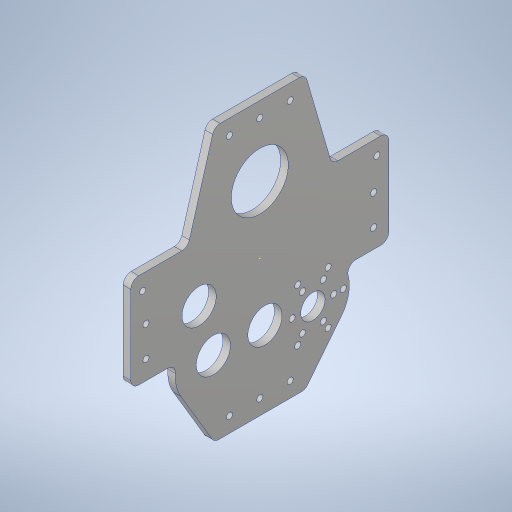
# Autodesk Inventor part: EL2-CGB-001
Saved by Autodesk Inventor 2023.4 (Build 274418000, 418)
## iProperties
Created: 2025-01-19
Part Number: EL2-CGB-001
Material: Aluminum 6061
Document SubType Name: Modeling
Designer: mavericks
Density: 2.7 g/cm^3
Appearance: Aluminum - Flat
Author: mavericks
Autodesk Inventor part; units mm, degrees
ref_plane "YZ Plane" through (0, 0, 0) normal (1, 0, 0) x (0, 1, 0)
ref_plane "XZ Plane" through (0, 0, 0) normal (0, 1, 0) x (-1, 0, 0)
ref_plane "XY Plane" through (0, 0, 0) normal (0, 0, 1) x (1, 0, 0)
sketch "Sketch1" plane through (0, 0, 0) normal (1, 0, 0) x (0, 1, 0)
  line L0 (114.3, 107.95) -> (-114.3, 107.95) construction
  line L1 (-114.3, 107.95) -> (-114.3, 82.55) construction
  line L2 (-114.3, 82.55) -> (114.3, 82.55) construction
  line L3 (114.3, 82.55) -> (114.3, 107.95) construction
  line L4 (-44.45, 128.7526) -> (-69.85, 128.7526) construction
  line L5 (-69.85, 128.7526) -> (-69.85, 79.4258) construction
  line L6 (-69.85, 79.4258) -> (-44.45, 79.4258) construction
  line L7 (-44.45, 79.4258) -> (-44.45, 128.7526) construction
  line L8 (69.85, 128.7526) -> (44.45, 128.7526) construction
  line L9 (44.45, 128.7526) -> (44.45, 79.4258) construction
  line L10 (44.45, 79.4258) -> (69.85, 79.4258) construction
  line L11 (69.85, 79.4258) -> (69.85, 128.7526) construction
  line L12 (44.45, 104.0892) -> (-44.45, 104.0892) construction
  line L13 (0, 0) -> (-27.2932, 0) construction
  line L14 (114.3, -107.95) -> (-114.3, -107.95) construction
  line L15 (-114.3, -107.95) -> (-114.3, -82.55) construction
  line L16 (-114.3, -82.55) -> (114.3, -82.55) construction
  line L17 (114.3, -82.55) -> (114.3, -107.95) construction
  line L18 (-44.45, -128.7526) -> (-69.85, -128.7526) construction
  line L19 (-69.85, -128.7526) -> (-69.85, -79.4258) construction
  line L20 (-69.85, -79.4258) -> (-44.45, -79.4258) construction
  line L21 (-44.45, -79.4258) -> (-44.45, -128.7526) construction
  line L22 (69.85, -128.7526) -> (44.45, -128.7526) construction
  line L23 (44.45, -128.7526) -> (44.45, -79.4258) construction
  line L24 (44.45, -79.4258) -> (69.85, -79.4258) construction
  line L25 (69.85, -79.4258) -> (69.85, -128.7526) construction
  line L26 (44.45, -104.0892) -> (-44.45, -104.0892) construction
  line L27 (114.3, 82.55) -> (88.9, 82.55) construction
  line L28 (88.9, 82.55) -> (88.9, -82.55) construction
  line L29 (88.9, -82.55) -> (114.3, -82.55) construction
  line L30 (114.3, -82.55) -> (114.3, 82.55) construction
  line L31 (-114.3, 82.55) -> (-88.9, 82.55) construction
  line L32 (-88.9, 82.55) -> (-88.9, -82.55) construction
  line L33 (-88.9, -82.55) -> (-114.3, -82.55) construction
  line L34 (-114.3, -82.55) -> (-114.3, 82.55) construction
  point P0 (0, 82.55)
  point P1 (0, 104.0892)
  point P2 (0, -82.55)
  point P3 (0, -104.0892)
  dimension "d0" = 228.6
  dimension "d1" = 25.4
  dimension "d2" = 82.55
  dimension "d3" = 25.4
  dimension "d4" = 49.3268
  dimension "d6" = 88.9
  dimension "d7" = 3.1242
  dimension "d8" = 25.4
  dimension "d9" = 25.4
  constraints: 70 end point, 16 symmetric about line, 12 parallel, 7 horizontal, 5 perpendicular, 4 midpoint, 2 vertical alignment, 1 horizontal alignment, 1 point on line
  measures "d0" distance of L2.end L1.end
  measures "d1" distance of L1.end L0.end
  measures "d2" vertical distance of L13.start L2.end
  measures "d3" distance of L6.end L5.end
  measures "d4" distance of L5.end L4.end
  measures "d6" distance of L4.start L8.end
  measures "d7" distance from line of L2 L6.end
  measures "d8" distance between parallel lines of L28 L30
  measures "d9" distance between parallel lines of L34 L32
sketch "Sketch2" plane through (0, 0, 0) normal (1, 0, 0) x (0, 1, 0)
  line L0 (-114.3, 107.95) -> (-114.3, 82.55) construction
  line L1 (44.45, 104.0892) -> (-44.45, 104.0892) construction
  line L2 (-114.3, 82.55) -> (114.3, 82.55) construction
  line L3 (114.3, 107.95) -> (-114.3, 107.95) construction
  line L4 (44.45, 79.4258) -> (69.85, 79.4258) construction
  line L5 (114.3, 82.55) -> (114.3, 107.95) construction
  line L6 (-69.85, 79.4258) -> (-44.45, 79.4258) construction
  line L7 (-44.45, 79.4258) -> (-44.45, 128.7526) construction
  line L8 (-69.85, 128.7526) -> (-69.85, 79.4258) construction
  line L9 (-44.45, 128.7526) -> (-69.85, 128.7526) construction
  line L10 (88.9, 82.55) -> (88.9, -82.55) construction
  line L11 (114.3, -82.55) -> (114.3, 82.55) construction
  line L12 (-114.3, -82.55) -> (114.3, -82.55) construction
  line L13 (114.3, -107.95) -> (-114.3, -107.95) construction
  line L14 (44.45, -104.0892) -> (-44.45, -104.0892) construction
  line L15 (-114.3, 82.55) -> (-88.9, 82.55) construction
  line L16 (-88.9, 82.55) -> (-88.9, -82.55) construction
  line L17 (-114.3, -82.55) -> (-114.3, 82.55) construction
  line L18 (-69.85, -79.4258) -> (-44.45, -79.4258) construction
  line L19 (-88.9, -82.55) -> (-114.3, -82.55) construction
  line L20 (-44.45, -79.4258) -> (-44.45, -128.7526) construction
  line L21 (-44.45, -128.7526) -> (-69.85, -128.7526) construction
  line L22 (-69.85, -128.7526) -> (-69.85, -79.4258) construction
  line L23 (-114.3, -107.95) -> (-114.3, -82.55) construction
  line L24 (44.45, -79.4258) -> (69.85, -79.4258) construction
  line L25 (44.45, -128.7526) -> (44.45, -79.4258) construction
  line L26 (88.9, -82.55) -> (114.3, -82.55) construction
  line L27 (69.85, -128.7526) -> (44.45, -128.7526) construction
  line L28 (69.85, -79.4258) -> (69.85, -128.7526) construction
  line L29 (114.3, -82.55) -> (114.3, -107.95) construction
  line L30 (69.85, 128.7526) -> (44.45, 128.7526) construction
  line L31 (44.45, 128.7526) -> (44.45, 79.4258) construction
  line L32 (69.85, 79.4258) -> (69.85, 128.7526) construction
  line L33 (114.3, 82.55) -> (88.9, 82.55) construction
  circle A0 centre (-57.15, -44.45) radius 6.35 construction
  circle A1 centre (-50.8, -4.3092) radius 34.29 construction
  circle A2 centre (-50.8, -4.3092) radius 11.43 construction
  circle A3 centre (-50.8, 38.8708) radius 31.75 construction
  circle A4 centre (-50.8, 38.8708) radius 15.24 construction
  circle A5 centre (-9.3005, 50.8) radius 27.94 construction
  circle A6 centre (-57.15, -44.45) radius 30.48 construction
  circle A7 centre (-57.15, -44.45) radius 10.16
  circle A8 centre (-50.8, -4.3092) radius 14.2875
  circle A9 centre (-50.8, 38.8708) radius 14.2875
  circle A10 centre (-9.3005, 50.8) radius 14.2875
  circle A11 centre (-9.3005, 50.8) radius 20.6375 construction
  circle A12 centre (-50.8, 38.8708) radius 20.6375 construction
  circle A13 centre (-50.8, -4.3092) radius 20.6375 construction
  circle A14 centre (-57.15, -44.45) radius 17.4625 construction
  circle A15 centre (-57.15, -44.45) radius 25.4 construction
  line L34 (-41.275, -131.9276) -> (-41.275, -76.2508) construction
  line L35 (-41.275, -76.2508) -> (-73.025, -76.2508) construction
  line L36 (-73.025, -76.2508) -> (-73.025, -131.9276) construction
  line L37 (-73.025, -131.9276) -> (-41.275, -131.9276) construction
  line L38 (-76.0619, -68.3533) -> (-114.3, -38.1)
  line L39 (-114.3, -38.1) -> (-114.3, 38.1)
  line L40 (-114.3, 38.1) -> (-41.275, 38.1) construction
  line L41 (-41.275, 38.1) -> (-41.275, 104.0892) construction
  arc A16 (-76.0619, -68.3533) -> (-41.275, -70.4695) centre (-57.15, -44.45) ccw
  circle A17 centre (55.7676, 0) radius 23.8125
  circle A18 centre (55.7676, 0) radius 33.3375 construction
  line L42 (37.9487, 60.325) -> (114.3, 38.1)
  line L43 (114.3, 38.1) -> (114.3, -38.1)
  line L44 (114.3, -38.1) -> (37.9487, -60.325)
  line L45 (37.9487, -60.325) -> (37.9487, -107.95)
  line L46 (37.9487, -107.95) -> (-41.275, -107.95)
  line L47 (-41.275, -107.95) -> (-41.275, -70.4695)
  line L48 (37.9487, 60.325) -> (37.9487, 107.95)
  line L49 (37.9487, 107.95) -> (-41.275, 107.95)
  circle A19 centre (-9.3005, 50.8) radius 20.6375 construction
  circle A20 centre (55.7676, 0) radius 57.277 construction
  line L50 (-41.275, 107.95) -> (-41.275, 69.1584)
  line L51 (-67.0064, 66.1731) -> (-114.3, 38.1)
  arc A21 (-41.275, 69.1584) -> (-67.0064, 66.1731) centre (-50.8, 38.8708) ccw
  point P0 (25.2487, 98.0186)
  point P1 (0, 95.25)
  point P2 (25.2487, -98.0186)
  point P3 (0, -95.25)
  point P4 (-25.4, -95.25)
  point P5 (-25.4, 95.25)
  point P6 (114.3, -95.25)
  point P7 (114.3, 95.25)
  point P8 (0, -82.55)
  point P9 (-101.6, 25.4)
  point P10 (-101.6, 0)
  point P11 (-101.6, -25.4)
  point P12 (-88.9, 0)
  point P13 (-101.6, 82.55)
  point P14 (-57.15, -19.05)
  point P15 (-57.15, -26.9875)
  point P16 (-79.147, -31.75)
  point P17 (-72.273, -35.7187)
  point P18 (-79.147, -57.15)
  point P19 (-72.273, -53.1812)
  point P20 (-57.15, -69.85)
  point P21 (-57.15, -61.9125)
  point P22 (-35.153, -57.15)
  point P23 (-42.027, -53.1813)
  point P24 (-35.153, -31.75)
  point P25 (-42.027, -35.7188)
  point P26 (44.45, 104.0892)
  point P27 (-114.3, 0)
  point P28 (-114.3, 0)
  point P29 (88.9, 0)
  point P30 (101.6, 25.4)
  point P31 (101.6, 0)
  point P32 (101.6, -25.4)
  point P33 (101.6, 82.55)
  point P34 (114.3, 0)
  dimension "d33" = 34.925
  dimension "d34" = 50.8
  dimension "d10" = 12.7
  dimension "d11" = 68.58
  dimension "d12" = 22.86
  dimension "d13" = 63.5
  dimension "d14" = 30.48
  dimension "d15" = 55.88
  dimension "d16" = 60.96
  dimension "d19" = 31.75
  dimension "d23" = 20.32
  dimension "d24" = 28.575
  dimension "d26" = 25.4
  dimension "d27" = 25.4
  dimension "d28" = 25.4
  dimension "d29" = 25.4
  dimension "d30" = 6.35
  dimension "d31" = 6.35
  dimension "d32" = 6.35
  dimension "d37" = 360
  dimension "d41" = 3.175
  dimension "d42" = 76.2
  dimension "d60" = 89.0513
  dimension "d63" = 38.1
  dimension "d64" = 38.1
  dimension "d66" = 38.1
  dimension "d67" = 31.75
  dimension "d68" = 47.625
  dimension "d70" = 9.525
  dimension "d71" = 47.625
  dimension "d73" = 82.55
  dimension "d74" = 12.7
  dimension "d75" = 41.275
  dimension "d76" = 114.554
  dimension "d78" = 9.9314
  dimension "d79" = 9.9314
  constraints: 36 end point, 20 centre point, 18 vertical alignment, 14 coincident, 11 horizontal alignment, 11 midpoint, 11 point on line, 8 point on circle, 5 tangent, 3 collinear, 2 equal radius, 2 perpendicular, 1 horizontal, 1 vertical, 20 other
  measures "d10" diameter of A0
  measures "d11" diameter of A1
  measures "d12" diameter of A2
  measures "d13" diameter of A3
  measures "d14" diameter of A4
  measures "d15" diameter of A5
  measures "d16" diameter of A6
  measures "d19" distance from line of L16 A0.centre
  measures "d23" diameter of A7
  measures "d24" diameter of A8
  measures "d26" distance of point (-25.4, 95.25) point (0, 95.25)
  measures "d27" distance of point (25.249, 98.019) point (0, 95.25)
  measures "d28" distance of point (-101.6, 0) point (-101.6, 25.4)
  measures "d29" distance of point (-101.6, 0) point (-101.6, -25.4)
  measures "d30" radial gap between concentric circles of A10 A11
  measures "d31" radial gap between concentric circles of A9 A12
  measures "d32" radial gap between concentric circles of A8 A13
  measures "d41" distance between parallel lines of L20 L34
  measures "d42" distance of L38.end L39.end
  measures "d60" distance from line of L5 point (25.249, 98.019)
  measures "d63" distance from line of L12 A0.centre
  measures "d64" distance from line of L16 A1.centre
  measures "d66" distance from line of L16 A3.centre
  measures "d67" distance from line of L2 A5.centre
  measures "d68" diameter of A17
  measures "d70" radial gap between concentric circles of A17 A18
  measures "d71" distance of L42.start L48.end
  measures "d73" distance of A17.centre A5.centre
  measures "d74" horizontal distance of point (25.249, 98.019) L48.end
  measures "d75" diameter of A19
  measures "d76" diameter of A20
  measures "d78" distance from line of point (25.249, 98.019) L3
  measures "d79" distance from line of L13 point (25.249, -98.019)
extrude "Extrusion1" add sketch "Sketch2" along normal blind 6.35
hole "Mount Holes" at (0, -88.9, 82.55) at (0, -114.3, 107.95) at (0, -69.85, 79.4258) at (0, -44.45, -79.4258) at (0, 44.45, -79.4258) at (0, 69.85, -79.4258) at (0, 44.45, -128.7526) at (0, 44.45, 128.7526) at (0, 25.2487, 98.0186) at (0, 0, 95.25) at (0, 25.2487, -98.0186) at (0, 0, -95.25) at (0, -25.4, -95.25) at (0, -25.4, 95.25) at (0, -101.6, 25.4) at (0, -101.6, 0) at (0, -101.6, -25.4) at (0, 101.6, 25.4) at (0, 101.6, 0) at (0, 101.6, -25.4) direction (1, 0, 0) diameter 5.1054 end through all clearance for "Flat Head Machine Screw (82)" size "#10" standard "Ansi Unified Screw Threads"
hole "Motor Mount Holes" at (0, -57.15, -26.9875) at (0, -79.147, -31.75) at (0, -72.273, -35.7187) at (0, -79.147, -57.15) at (0, -72.273, -53.1812) at (0, -57.15, -69.85) at (0, -57.15, -61.9125) at (0, -35.153, -57.15) at (0, -42.027, -53.1813) at (0, -35.153, -31.75) at (0, -42.027, -35.7188) direction (1, 0, 0) diameter 5.1054 end through all clearance for "Flat Head Machine Screw (82)" size "#10" standard "Ansi Unified Screw Threads"
sketch "Sketch3" plane through (6.35, 0, 0) normal (1, 0, 0) x (0, 0, -1)
  point P0 (0, 0)
fillet "Fillet1" radius 6.604 12 edges at (3.175, -41.275, 107.95) (3.175, -114.3, 38.1) (3.175, -114.3, -38.1) (3.175, -41.275, -70.4695) (3.175, -41.275, -107.95) (3.175, 37.9487, -107.95) (3.175, 37.9487, -60.325) (3.175, 114.3, -38.1) (3.175, 114.3, 38.1) (3.175, 37.9487, 60.325) (3.175, 37.9487, 107.95) (3.175, -41.275, 69.1584)
body "Solid1"
